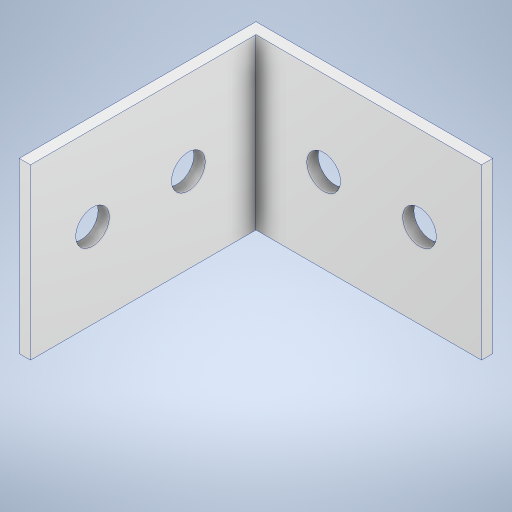
# Autodesk Inventor part: 3030_L-Bracket
Saved by Autodesk Inventor 2024 (Build 280153000, 153)
## iProperties
Created: 2025-12-17
Part Number: 3030_L-Bracket
Material: Aluminum 6061
Document SubType Name: Modeling
Designer: schar
Density: 2.7 g/cm^3
Appearance: Aluminum - Flat
Author: schar
Autodesk Inventor part; units mm, degrees
ref_plane "YZ Plane" through (0, 0, 0) normal (1, 0, 0) x (0, 1, 0)
ref_plane "XZ Plane" through (0, 0, 0) normal (0, 1, 0) x (-1, 0, 0)
ref_plane "XY Plane" through (0, 0, 0) normal (0, 0, 1) x (1, 0, 0)
sketch "Sketch1" plane through (0, 0, 0) normal (0, 1, 0) x (-1, 0, 0)
  line L0 (0, 0) -> (-2, 0)
  line L1 (-2, 0) -> (-2, 40)
  line L2 (-2, 40) -> (0, 40)
  line L3 (0, 40) -> (0, 0)
  line L4 (0, 0) -> (-42, 0)
  line L5 (-42, 0) -> (-42, -2)
  line L6 (-42, -2) -> (0, -2)
  line L7 (0, -2) -> (0, 0)
  dimension "d0" = 2
  dimension "d1" = 40
  dimension "d2" = 42
  dimension "d3" = 2
  constraints: 16 end point, 4 parallel, 2 horizontal, 2 perpendicular
  measures "d0" distance of L1.end L2.end
  measures "d1" distance of L0.end L1.end
  measures "d2" distance of L6.end L5.end
  measures "d3" distance of L5.end L4.end
extrude "Extrusion1" add sketch "Sketch1" along normal blind 30
sketch "Sketch2" plane through (2, 0, 0) normal (0, 0, 1) x (1, 0, 0)
  line L0 (40.0406, 0) -> (40, 14.9999)
  line L1 (40, 0) -> (40, 30) projected
  line L2 (40, 14.9999) -> (29, 14.9702)
  line L3 (29, 14.9702) -> (12.0001, 14.9242)
  point P0 (-2, 0)
  dimension "d6" = 15
  dimension "d7" = 11
  dimension "d8" = 17
  constraints: 6 end point, 2 coincident, 2 point on line, 1 perpendicular
  measures "d6" distance of L0.start L0.end
  measures "d7" distance of L0.end L2.end
  measures "d8" distance of L2.end L3.end
hole "Hole1" at (31, 14.9702, 0) at (14.0001, 14.9242, 0) direction (0, 0, -1) diameter 6 end through all
sketch "Sketch3" plane through (2, 0, 40) normal (1, 0, 0) x (0, 0, -1)
  line L0 (0, 0) -> (0, 30) projected
  line L1 (0, 0) -> (0, 15)
  line L2 (0, 15) -> (11, 15)
  line L3 (11, 15) -> (28, 15)
  point P0 (40, 0)
  dimension "d16" = 15
  dimension "d17" = 11
  dimension "d18" = 17
  constraints: 6 end point, 1 midpoint, 1 perpendicular, 1 point on line
  measures "d16" distance of L0.start L1.end
  measures "d17" distance of L1.end L2.end
  measures "d18" distance of L2.end L3.end
hole "Hole2" at (2, 15, 29) at (2, 15, 12) direction (-1, 0, 0) diameter 6 end through all
body "Solid1"
